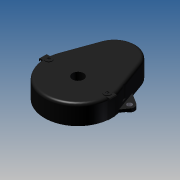
# Autodesk Inventor part: Stepper Motor SAIA Reducer31082011
Saved by Autodesk Inventor 2012 SP1 (Build 160190100, 190)
## iProperties
Shininess: 64.0
Length Units: 11269
Angle Units: 11279
Time Units: 11290
Mass Units: 11283
Length Display Precision: 3
Angle Display Precision: 2
Compacted: True
Part Number: Stepper Motor SAIA Reducer31082011
Document SubType Name: Modeling
Created: 2004-06-12
Designer: flg
Density: 1 g/cm^3
Material: Fourniture / Geliefertes
Description: Réducteur SAIA direction
Density: 0.0
Volumn: 0.0
Area: 0.0
PropertySet Name: Model Information
Control State: 0
Master: False
Checked Out: False
Author: flg
Autodesk Inventor part; units mm, degrees
ref_plane "YZ Plane" through (0, 0, 0) normal (1, 0, 0) x (0, 1, 0)
ref_plane "XZ Plane" through (0, 0, 0) normal (0, 1, 0) x (-1, 0, 0)
ref_plane "XY Plane" through (0, 0, 0) normal (0, 0, 1) x (1, 0, 0)
sketch "Sketch1" plane through (0, 0, 0) normal (0, 0, 1) x (1, 0, 0)
  arc A0 (-22.5835, 8.1231) -> (22.5835, 8.1231) centre (0, 0) ccw
  arc A1 (14.3029, 31.1446) -> (-14.3029, 31.1446) centre (0, 26) ccw
  line L0 (0, 0) -> (0, -24) construction
  line L1 (0, 0) -> (0, 41.2) construction
  line L2 (-22.5835, 8.1231) -> (-14.3029, 31.1446)
  line L3 (14.3029, 31.1446) -> (22.5835, 8.1231)
  dimension "d0" = 48
  dimension "d28" = 30.4
  dimension "d37" = 26
  constraints: 8 end point, 6 point on circle, 4 tangent, 2 centre point, 1 collinear, 1 point on line, 1 vertical, 1 other
  measures "d0" diameter of A0
  measures "d28" diameter of A1
  measures "d37" distance of L0.start A1.centre
extrude "Extrusion1" add sketch "Sketch1" along normal blind 14
fillet "Fillet1" radius 2 4 edges at (0, -24, 14) (-18.4432, 19.6338, 14) (0, 41.2, 14) (18.4432, 19.6338, 14)
sketch "Sketch2" plane through (0, 0, 0) normal (0, 0, -1) x (-1, 0, 0)
  arc A0 (14.3029, 31.1446) -> (-14.3029, 31.1446) centre (0, 26) ccw construction
  arc A1 (-22.5835, 8.1231) -> (22.5835, 8.1231) centre (0, 0) ccw construction
  line L0 (14.3029, 31.1446) -> (22.5835, 8.1231) construction
  arc A2 (14.3029, 31.1446) -> (-14.3029, 31.1446) centre (0, 26) ccw construction
  line L1 (-22.5835, 8.1231) -> (-14.3029, 31.1446) construction
  arc A3 (-22.5835, 8.1231) -> (22.5835, 8.1231) centre (0, 0) ccw construction
  line L2 (14.3029, 31.1446) -> (22.5835, 8.1231) construction
  line L3 (0, -37.04) -> (0, 54.24) construction
  line L4 (-38.297, 0) -> (34.3828, 0) construction
  circle A4 centre (-24, 13) radius 1.75
  arc A5 (-25.8797, 15.9524) -> (-26.8309, 10.9418) centre (-24, 13) ccw
  line L5 (-26.8309, 10.9418) -> (-23.2379, 6)
  line L6 (-17.9518, 21) -> (-22.5835, 8.1231)
  arc A6 (-22.5835, 8.1231) -> (-23.2379, 6) centre (0, 0) ccw
  line L7 (-25.8797, 15.9524) -> (-17.9518, 21)
  dimension "d6" = 3.5
  dimension "d7" = 7
  dimension "d8" = 13
  dimension "d9" = 24
  dimension "d54" = 6
  dimension "d55" = 21
  constraints: 6 end point, 6 point on circle, 5 tangent, 3 centre point, 1 coincident, 1 concentric, 1 point on line
  measures "d6" diameter of A4
  measures "d7" diameter of A5
  measures "d8" distance from line of L4 A4.centre
  measures "d9" distance from line of L3 A4.centre
  measures "d54" distance from line of L4 L5.end
  measures "d55" distance from line of L4 L6.start
extrude "Extrusion2" add sketch "Sketch2" against normal blind 2
mirror "Mirror1" about plane through (0, 0, 0) normal (1, 0, 0) of "Extrusion2"
sketch "Sketch3" plane through (0, 0, 0) normal (0, 0, -1) x (-1, 0, 0)
  circle A0 centre (-24, 13) radius 1.75 construction
  circle A1 centre (24, 13) radius 1.75 construction
  line L0 (-24, 13) -> (24, 13) construction
  circle A2 centre (0, 26) radius 4
  dimension "d29" = 13
  dimension "d30" = 8
  constraints: 2 end point, 1 centre point, 1 horizontal
  measures "d29" distance from line of L0 A2.centre
  measures "d30" diameter of A2
extrude "Extrusion3" add sketch "Sketch3" along normal blind 2
sketch "Sketch5" plane through (0, 0, 14) normal (0, 0, 1) x (1, 0, 0)
  line L0 (0, 0) -> (27.3766, 0) construction
  arc A0 (-20.7016, 7.4462) -> (20.7016, 7.4462) centre (0, 0) ccw construction
  line L1 (21.857, 2.5044) -> (25.5, 2.5044)
  line L2 (21.857, -2.5044) -> (25.5, -2.5044)
  line L3 (25.5, 2.5044) -> (25.5, -2.5044)
  arc A1 (21.857, -2.5044) -> (21.857, 2.5044) centre (0, 0) ccw
  dimension "d20" = 25.5
  constraints: 8 end point, 3 point on circle, 2 symmetric about line, 1 centre point, 1 horizontal, 1 parallel, 1 perpendicular
  measures "d20" distance from line of L3 L0.start
extrude "Extrusion5" add sketch "Sketch5" against normal up to surface (14 mm away)
sketch "Sketch6" plane through (21.857, -2.5044, 14) normal (0, -1, 0) x (1, 0, 0)
  line L0 (3.643, 0) -> (3.643, -14) construction
  line L1 (3.643, -14) -> (2.012, -14) construction
  line L2 (2.212, -14) -> (2.212, -1)
  line L3 (2.212, -1) -> (2.779, -1)
  line L4 (2.779, -1) -> (3.143, -2)
  line L5 (3.143, -2) -> (3.643, -2)
  line L6 (3.643, -2) -> (3.643, -14)
  line L7 (3.643, -14) -> (2.212, -14)
  line L8 (0, 0) -> (3.643, 0) construction
  point P0 (-21.857, -14)
  dimension "d21" = 0.2
  dimension "d22" = 2
  dimension "d23" = 0.5
  dimension "d24" = 1
  dimension "d25" = 110
  constraints: 12 end point, 3 perpendicular, 2 collinear, 2 point on line
  measures "d21" distance from line of L2 L1.end
  measures "d22" distance between parallel lines of L8 L5
  measures "d23" distance of L4.end L5.end
  measures "d24" distance between parallel lines of L8 L3
  measures "d25" angle of L4 L5
extrude "Extrusion6" cut sketch "Sketch6" against normal up to surface (5.0089 mm away)
mirror "Mirror2" about plane through (0, 0, 0) normal (1, 0, 0) of "Extrusion5", "Extrusion6"
sketch "Sketch7" plane through (0, 26, -2) normal (0, 0, -1) x (-1, 0, 0)
  circle A0 centre (0, 0) radius 4 construction
  circle A1 centre (0, 0) radius 2
  point P0 (0, -26)
  dimension "d31" = 4
  constraints: 1 centre point, 1 coincident
  measures "d31" diameter of A1
extrude "Extrusion7" add sketch "Sketch7" along normal blind 10
chamfer "Chamfer1" distance 0.5 angle 45 2 edges at (-25.5, 0, 14) (25.5, 0, 14)
sketch "Sketch8" plane through (0, 0, 14) normal (0, 0, 1) x (1, 0, 0)
  line L0 (0, 0) -> (21, 0) construction
  line L1 (0, 0) -> (0, 4.6027) construction
  point P0 (-21, 0)
  point P1 (-21, 0)
  dimension "d45" = 42
  constraints: 4 end point, 2 coincident, 2 symmetric about line, 1 horizontal, 1 perpendicular
  measures "d45" distance of L0.end point (-21, 0)
hole "Hole2" at (21, 0, 14) at (-21, 0, 14) direction (0, 0, -1) diameter 2.013 depth 8 tip angle 118 thread size "M2.5x0.45" class "6H" standard "ISO Metric profile"
sketch "Sketch10" plane through (0, 0, 14) normal (0, 0, 1) x (1, 0, 0)
  circle A0 centre (-24, 13) radius 1.75 construction
  circle A1 centre (-24, 13) radius 3.5 construction
  line L0 (-22.6035, 16.2093) -> (-24.3099, 16.9519)
  line L1 (-23.6047, 9.5224) -> (-25.6314, 9.292)
  line L2 (-17.9518, 21) -> (-25.8797, 15.9524) construction
  line L3 (-26.8309, 10.9418) -> (-23.2379, 6) construction
  line L4 (-24.3099, 16.9519) -> (-25.8797, 15.9524)
  line L5 (-25.6314, 9.292) -> (-26.8309, 10.9418)
  arc A2 (-23.6047, 9.5224) -> (-22.6035, 16.2093) centre (-24, 13) ccw
  arc A3 (-25.8797, 15.9524) -> (-26.8309, 10.9418) centre (-24, 13) ccw
  point P0 (0, 0)
  dimension "d58" = 7
  dimension "d62" = 30
  dimension "d63" = 56
  constraints: 8 end point, 6 point on circle, 4 tangent, 3 centre point, 2 coincident, 2 collinear, 2 point on line
  measures "d58" diameter of A1
  measures "d62" angle of L1 L0
  measures "d63" angle of L2 L0
extrude "Extrusion9" cut sketch "Sketch10" against normal blind 10
mirror "Mirror3" about plane through (0, 0, 0) normal (1, 0, 0) of "Extrusion9"
sketch "Sketch12" plane through (0, 0, 14) normal (0, 0, 1) x (1, 0, 0)
  circle A0 centre (-21, 0) radius 1.0065 construction
  circle A1 centre (21, 0) radius 1.0065 construction
  line L0 (25, 2.5044) -> (25, -2.5044) construction
  line L1 (21.857, 2.5044) -> (25, 2.5044) construction
  arc A2 (21.857, 2.5044) -> (20.7016, 7.4462) centre (0, 0) ccw construction
  line L2 (12.4209, 30.4677) -> (20.7016, 7.4462) construction
  arc A3 (12.4209, 30.4677) -> (-12.4209, 30.4677) centre (0, 26) ccw construction
  line L3 (-20.7016, 7.4462) -> (-12.4209, 30.4677) construction
  arc A4 (-20.7016, 7.4462) -> (-21.857, 2.5044) centre (0, 0) ccw construction
  line L4 (-21.857, 2.5044) -> (-25, 2.5044) construction
  line L5 (-25, -2.5044) -> (-25, 2.5044) construction
  line L6 (-25, -2.5044) -> (-21.857, -2.5044) construction
  arc A5 (-21.857, -2.5044) -> (21.857, -2.5044) centre (0, 0) ccw construction
  line L7 (25, -2.5044) -> (21.857, -2.5044) construction
  line L8 (-21, 0) -> (21, 0) construction
  circle A6 centre (0, 0) radius 4
  dimension "d68" = 8
  constraints: 2 end point, 1 centre point, 1 coincident, 1 parallel
  measures "d68" diameter of A6
extrude "Extrusion11" cut sketch "Sketch12" against normal blind 6
sketch "Sketch14" plane through (0, 0, 0) normal (0, 0, -1) x (-1, 0, 0)
  line L0 (24.069, -2.5044) -> (24.069, 2.5044) construction
  line L1 (23.869, 2.5044) -> (24.069, 2.5044) construction
  arc A0 (23.869, 2.5044) -> (23.2379, 6) centre (0, 0) ccw construction
  line L2 (26.8309, 10.9418) -> (23.2379, 6) construction
  arc A1 (26.8309, 10.9418) -> (25.8797, 15.9524) centre (24, 13) ccw construction
  line L3 (17.9518, 21) -> (25.8797, 15.9524) construction
  line L4 (14.3029, 31.1446) -> (17.9518, 21) construction
  arc A2 (14.3029, 31.1446) -> (-14.3029, 31.1446) centre (0, 26) ccw construction
  line L5 (-17.9518, 21) -> (-14.3029, 31.1446) construction
  line L6 (-17.9518, 21) -> (-25.8797, 15.9524) construction
  arc A3 (-25.8797, 15.9524) -> (-26.8309, 10.9418) centre (-24, 13) ccw construction
  line L7 (-26.8309, 10.9418) -> (-23.2379, 6) construction
  arc A4 (-23.2379, 6) -> (-23.869, 2.5044) centre (0, 0) ccw construction
  line L8 (-23.869, 2.5044) -> (-24.069, 2.5044) construction
  line L9 (-24.069, 2.5044) -> (-24.069, -2.5044) construction
  line L10 (-24.069, -2.5044) -> (-23.869, -2.5044) construction
  arc A5 (-23.869, -2.5044) -> (23.869, -2.5044) centre (0, 0) ccw construction
  line L11 (24.069, -2.5044) -> (23.869, -2.5044) construction
  circle A6 centre (-24, 13) radius 1.75 construction
  circle A7 centre (24, 13) radius 1.75 construction
  circle A8 centre (0, 26) radius 4 construction
  circle A9 centre (-24, 13) radius 3.5
  circle A10 centre (-24, 13) radius 1.75
  circle A11 centre (24, 13) radius 1.75
  circle A12 centre (24, 13) radius 3.5
  constraints: 4 centre point, 4 coincident, 2 concentric
extrude "Extrusion12" add sketch "Sketch14" along normal blind 0.5
sketch "Sketch15" plane through (0, 0, 14) normal (0, 0, 1) x (1, 0, 0)
  circle A0 centre (0, 0) radius 4 construction
  circle A1 centre (-21, 0) radius 1.0065 construction
  circle A2 centre (21, 0) radius 1.0065 construction
  line L0 (25, 2.5044) -> (25, -2.5044) construction
  line L1 (21.857, 2.5044) -> (25, 2.5044) construction
  arc A3 (21.857, 2.5044) -> (20.7016, 7.4462) centre (0, 0) ccw construction
  line L2 (12.4209, 30.4677) -> (20.7016, 7.4462) construction
  arc A4 (12.4209, 30.4677) -> (-12.4209, 30.4677) centre (0, 26) ccw construction
  line L3 (-20.7016, 7.4462) -> (-12.4209, 30.4677) construction
  arc A5 (-20.7016, 7.4462) -> (-21.857, 2.5044) centre (0, 0) ccw construction
  line L4 (-21.857, 2.5044) -> (-25, 2.5044) construction
  line L5 (-25, -2.5044) -> (-25, 2.5044) construction
  line L6 (-25, -2.5044) -> (-21.857, -2.5044) construction
  arc A6 (-21.857, -2.5044) -> (21.857, -2.5044) centre (0, 0) ccw construction
  line L7 (25, -2.5044) -> (21.857, -2.5044) construction
  circle A7 centre (-21, 0) radius 1.0065
  circle A8 centre (-21, 0) radius 2.5
  circle A9 centre (21, 0) radius 1.0065
  circle A10 centre (21, 0) radius 2.5
  dimension "d73" = 5
  dimension "d74" = 5
  constraints: 4 centre point, 4 coincident, 2 concentric
  measures "d73" diameter of A8
  measures "d74" diameter of A10
extrude "Extrusion13" add sketch "Sketch15" along normal blind 0.4
body "Solid1"
